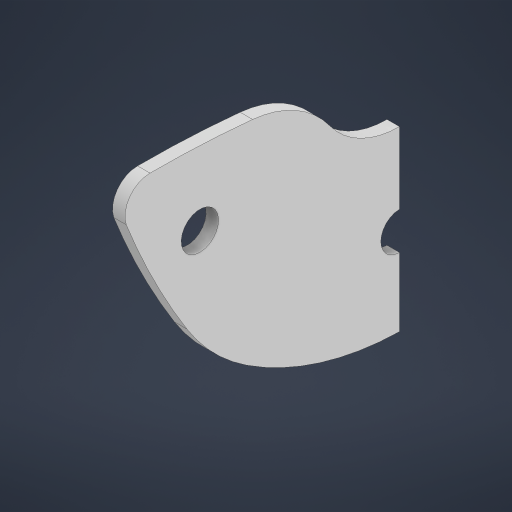
# Autodesk Inventor part: sled-inner
Saved by Autodesk Inventor 2024 (Build 280153000, 153)
## iProperties
Created: 2024-01-29
Part Number: sled-inner
Material: Generic
Document SubType Name: Modeling
Designer: macbook
Density: 1 g/cm^3
Appearance: Default
Author: macbook
Autodesk Inventor part; units mm, degrees
ref_plane "YZ Plane" through (0, 0, 0) normal (1, 0, 0) x (0, 1, 0)
ref_plane "XZ Plane" through (0, 0, 0) normal (0, 1, 0) x (-1, 0, 0)
ref_plane "XY Plane" through (0, 0, 0) normal (0, 0, 1) x (1, 0, 0)
sketch "Sketch1" plane through (0, 6.2481, 6.7374) normal (1, 0, 0) x (0, 1, 0)
  line L0 (21.1383, 36.7567) -> (20.6141, 36.7567)
  arc A0 (24.3907, 33.5692) -> (18.0407, 33.5826) centre (21.2157, 33.5826) ccw
  arc A1 (14.8657, -15.4374) -> (16.4404, -11.3937) centre (-103.5619, 33.0092) ccw
  arc A2 (18.4214, -5.6206) -> (14.8657, -28.6257) centre (91.0657, -28.6257) ccw
  arc A3 (20.207, 36.5931) -> (4.8725, 28.8882) centre (54.3249, -50.4207) ccw
  arc A4 (18.4214, -5.6206) -> (24.3907, 33.5692) centre (-103.5619, 33.0092) ccw
  line L1 (14.8657, 1.8326) -> (14.8657, 27.2326)
  line L2 (14.8657, 1.8326) -> (14.8657, 33.5826)
  line L3 (-10.5343, 1.8326) -> (14.8657, 1.8326) construction
  line L4 (-10.5343, 1.8326) -> (-10.5343, 27.2326)
  line L5 (-10.5343, 1.8326) -> (-23.2343, 1.8326)
  line L6 (-10.5343, 1.8326) -> (-10.5395, -10.8674)
  line L7 (-10.5395, -10.8674) -> (2.1605, -10.8727)
  line L8 (21.2157, 33.5826) -> (19.8929, 33.5826)
  line L9 (14.8657, 33.5826) -> (21.2157, 33.5826)
  arc A5 (-6.7994, 20.2847) -> (-12.9991, 12.2415) centre (9.812, 1.0696) ccw
  line L10 (14.8657, 33.5826) -> (-10.5343, 33.5826)
  line L11 (2.1605, -10.8727) -> (2.1605, -17.9797)
  line L12 (2.1605, -17.9797) -> (10.4725, -17.9797)
  line L13 (2.1605, -17.9797) -> (-5.7795, -17.9797)
  line L14 (-8.9545, -14.8047) -> (-8.9545, 1.0703)
  line L15 (13.6475, -14.8047) -> (13.6475, 1.8326)
  arc A6 (-2.9466, 21.2359) -> (-8.9545, 1.0703) centre (27.8921, 1.0703) ccw
  arc A7 (4.8725, 28.8882) -> (-2.9466, 21.2359) centre (18.3119, 7.3349) ccw
  arc A8 (16.4403, 9.623) -> (23.7808, 20.5184) centre (10.0212, 21.8681) ccw
  arc A9 (18.1559, 10.6889) -> (13.6475, 1.8326) centre (24.6004, 1.8326) ccw
  arc A10 (10.4725, -17.9797) -> (13.6475, -14.8047) centre (10.4725, -14.8047) ccw
  arc A11 (-8.9545, -14.8047) -> (-5.7795, -17.9797) centre (-5.7795, -14.8047) ccw
  line L16 (2.1605, -10.8727) -> (2.1605, 1.8273)
  line L17 (13.6475, 1.8326) -> (-8.9467, 1.8326)
  point P0 (0, 0)
  point P1 (13.6475, -17.9797)
  point P2 (-8.9545, -17.9797)
  point P3 (-8.9545, -10.868)
  point P4 (19.8992, 36.4718)
  dimension "d9" = 25.4
  dimension "d7" = 12.7
  dimension "d11" = 6.35
  dimension "d12" = 6.35
  dimension "d8" = 31.75
  dimension "d10" = 25.4
  dimension "d5" = 25.4
  dimension "d6" = 12.7
  dimension "d4" = 25.4
  dimension "d3" = 19.05
  dimension "d2" = 25.4
  dimension "d1" = 3.175
  dimension "d0" = 12.7
  constraints: 36 end point, 32 point on circle, 12 centre point, 12 tangent, 8 point on line, 5 horizontal, 5 vertical, 4 coincident, 3 perpendicular, 1 equal radius, 1 midpoint
  measures "d9" distance of L3.start L1.start
  measures "d7" distance of L3.start L5.end
  measures "d11" distance of L2.end L9.end
  measures "d12" diameter of A0
  measures "d8" distance of L1.start L2.end
  measures "d10" distance of L3.start L4.end
  measures "d5" radius of A5
  measures "d6" distance of L3.start L6.end
  measures "d4" distance of L2.end L10.end
  measures "d3" distance of point (-8.955, -17.98) L14.end
  measures "d2" radius of A7
  measures "d1" radius of A10
  measures "d0" distance of L11.start L16.end
extrude "Extrusion1" add sketch "Sketch1" along normal blind 1.5875 contours A4 A8 A9 L1 L2 L9 A0 A3 | A0 L9 L10 A3 | A9 L17 A6 A7 A3 L10 L2 L1
hole "Hole1" at (0, 21.1138, 33.9701) at (0, 8.4085, -4.1352) at (0, 8.4085, 8.5648) direction (1, 0, 0) diameter 4.7625 end through all
body "Solid1"
